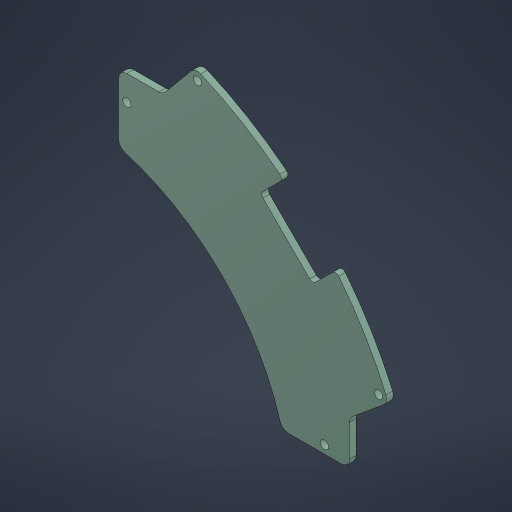
# Autodesk Inventor part: MotorDriver_PCB
Saved by Autodesk Inventor 2024.2 (Build 282272000, 272)
## iProperties
Created: 2023-12-22
Part Number: MotorDriver_PCB
Material: 一般
Document SubType Name: Modeling
Designer: Hanaoka
Density: 1 g/cm^3
Appearance: 既定
Author: Hanaoka
Autodesk Inventor part; units mm, degrees
ref_plane "YZ Plane" through (0, 0, 0) normal (1, 0, 0) x (0, 1, 0)
ref_plane "XZ Plane" through (0, 0, 0) normal (0, 1, 0) x (-1, 0, 0)
ref_plane "XY Plane" through (0, 0, 0) normal (0, 0, 1) x (1, 0, 0)
sketch "スケッチ1" plane through (0, 0, 0) normal (0, 0, 1) x (1, 0, 0)
  line L0 (54, -47.9205) -> (54, -40.1498) projected
  arc A0 (54.7258, -38.6082) -> (54, -40.1498) centre (56, -40.1498) ccw projected
  line L1 (54.7258, -38.6082) -> (62.3004, -32.3475) projected
  arc A1 (62.3004, -32.3475) -> (62.8611, -30.0103) centre (61.0262, -30.8059) ccw projected
  arc A2 (62.8611, -30.0103) -> (17.9102, 14.9406) centre (-16.5, -64.4205) ccw projected
  arc A3 (17.9102, 14.9406) -> (15.573, 14.3799) centre (17.1146, 13.1057) ccw projected
  line L2 (15.573, 14.3799) -> (9.3123, 6.8053) projected
  arc A4 (7.7707, 6.0795) -> (9.3123, 6.8053) centre (7.7707, 8.0795) ccw projected
  line L3 (7.7707, 6.0795) -> (0, 6.0795) projected
  arc A5 (0, 6.0795) -> (-2, 4.0795) centre (0, 4.0795) ccw projected
  line L4 (-2, 4.0795) -> (-2, -8.817) projected
  arc A6 (-2, -8.817) -> (-0.569, -10.7343) centre (0, -8.817) ccw projected
  arc A7 (37.1861, -48.4895) -> (-0.569, -10.7343) centre (-16.5, -64.4205) ccw projected
  arc A8 (37.1861, -48.4895) -> (39.1035, -49.9205) centre (39.1035, -47.9205) ccw projected
  line L5 (39.1035, -49.9205) -> (52, -49.9205) projected
  arc A9 (52, -49.9205) -> (54, -47.9205) centre (52, -47.9205) ccw projected
  circle A10 centre (47.9205, -47.9205) radius 1 projected
  circle A11 centre (0, 0) radius 1 projected
  circle A12 centre (17.1146, 13.1057) radius 1 projected
  circle A13 centre (61.0262, -30.8059) radius 1 projected
  point P0 (0, 0)
extrude "押し出し1" add sketch "スケッチ1" along normal blind 1.6
sketch "スケッチ2" plane through (0, 0, 1.6) normal (0, 0, 1) x (1, 0, 0)
  arc A0 (37.1861, -48.4895) -> (-0.569, -10.7343) centre (-16.5, -64.4205) ccw projected
  arc A1 (47.8768, -47.7509) -> (0, 0) centre (-16.5, -64.4205) ccw
  constraints: 2 point on circle, 1 centre point, 1 coincident
sketch "スケッチ3" plane through (0, 0, 1.6) normal (0, 0, 1) x (1, 0, 0)
  circle A0 centre (42.5969, -6.8792) radius 0.375 projected
  circle A1 centre (45.4254, -9.7076) radius 0.375 projected
  circle A2 centre (38.3543, -2.6366) radius 0.375 projected
  circle A3 centre (36.9401, -4.0508) radius 0.375 projected
  circle A4 centre (44.0111, -11.1218) radius 0.375 projected
  circle A5 centre (42.5969, -9.7076) radius 0.375 projected
  circle A6 centre (41.1827, -8.2934) radius 0.375 projected
  circle A7 centre (39.7685, -6.8792) radius 0.375 projected
  circle A8 centre (38.3543, -5.465) radius 0.375 projected
  circle A9 centre (44.0111, -8.2934) radius 0.375 projected
  circle A10 centre (39.7685, -4.0508) radius 0.375 projected
  circle A11 centre (41.1827, -5.465) radius 0.375 projected
  line L0 (39.1035, -49.9205) -> (52, -49.9205) projected
  arc A12 (52, -49.9205) -> (54, -47.9205) centre (52, -47.9205) ccw projected
  line L1 (54, -47.9205) -> (54, -40.1498) projected
  arc A13 (54.7258, -38.6082) -> (54, -40.1498) centre (56, -40.1498) ccw projected
  line L2 (54.7258, -38.6082) -> (62.3004, -32.3475) projected
  arc A14 (62.3004, -32.3475) -> (62.8611, -30.0103) centre (61.0262, -30.8059) ccw projected
  arc A15 (62.8611, -30.0103) -> (17.9102, 14.9406) centre (-16.5, -64.4205) ccw projected
  arc A16 (17.9102, 14.9406) -> (15.573, 14.3799) centre (17.1146, 13.1057) ccw projected
  line L3 (15.573, 14.3799) -> (9.3123, 6.8053) projected
  arc A17 (7.7707, 6.0795) -> (9.3123, 6.8053) centre (7.7707, 8.0795) ccw projected
  line L4 (7.7707, 6.0795) -> (0, 6.0795) projected
  arc A18 (0, 6.0795) -> (-2, 4.0795) centre (0, 4.0795) ccw projected
  line L5 (-2, 4.0795) -> (-2, -8.817) projected
  arc A19 (-2, -8.817) -> (-0.569, -10.7343) centre (0, -8.817) ccw projected
  arc A20 (37.1861, -48.4895) -> (-0.569, -10.7343) centre (-16.5, -64.4205) ccw projected
  arc A21 (37.1861, -48.4895) -> (39.1035, -49.9205) centre (39.1035, -47.9205) ccw projected
  circle A22 centre (17.1146, 13.1057) radius 1 projected
  circle A23 centre (61.0262, -30.8059) radius 1 projected
  circle A24 centre (0, 0) radius 1 projected
  circle A25 centre (47.9205, -47.9205) radius 1 projected
  line L6 (44.6647, -3.2558) -> (23.098, -24.8225) construction
  line L7 (50.6967, -9.9517) -> (45.0399, -15.6085)
  line L8 (45.0399, -15.6085) -> (32.3119, -2.8806)
  line L9 (32.3119, -2.8806) -> (37.9688, 2.7762)
  arc A26 (62.8611, -30.0103) -> (17.9102, 14.9406) centre (-16.5, -64.4205) ccw projected
  point P0 (0, 0)
  dimension "d2" = 18
  dimension "d3" = 8
  constraints: 8 end point, 4 point on circle, 3 parallel, 1 perpendicular
  measures "d2" distance of L7.end L8.end
  measures "d3" distance of L8.end L9.end
extrude "押し出し2" cut sketch "スケッチ3" against normal up to surface (1.6 mm away) contours A0 | A1 | A2 | A3 | A4 | A5 | A6 | A7 | A8 | A9 | A10 | A11 | L7 L8 L9 A15
fillet "フィレット1" radius 1 4 edges at (50.6967, -9.9517, 0.8) (45.0399, -15.6085, 0.8) (32.3119, -2.8806, 0.8) (37.9688, 2.7762, 0.8)
